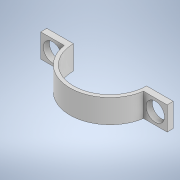
# Autodesk Inventor part: clamphalf
Saved by Autodesk Inventor 2020.2 (Build 242310000, 310)
## iProperties
Created: 2020-02-20
Part Number: clamphalf
Material: Generic
Document SubType Name: Modeling
Designer: ColinP
Density: 1 g/cm^3
Appearance: Default
Author: ColinP
Autodesk Inventor part; units mm, degrees
ref_plane "YZ Plane" through (0, 0, 0) normal (1, 0, 0) x (0, 1, 0)
ref_plane "XZ Plane" through (0, 0, 0) normal (0, 1, 0) x (-1, 0, 0)
ref_plane "XY Plane" through (0, 0, 0) normal (0, 0, 1) x (1, 0, 0)
sketch "Sketch1" plane through (0, 0, 0) normal (0, 1, 0) x (-1, 0, 0)
  circle A0 centre (0, 0) radius 7.75
  circle A1 centre (0, 0) radius 8.5
  line L0 (8.5, 0) -> (7.75, 0)
  line L1 (-7.75, 0) -> (-8.5, 0)
  line L2 (8.5, 0) -> (8.4, 0)
  line L3 (8.4, 0) -> (8.4, 1.3)
  line L4 (8.4, 1.3) -> (13.4, 1.3)
  line L5 (13.4, 1.3) -> (13.4, 0)
  line L6 (13.4, 0) -> (8.5, 0)
  line L7 (-8.5, 0) -> (-8.4, 0)
  line L8 (-8.4, 0) -> (-8.4, 1.3)
  line L9 (-8.4, 1.3) -> (-13.4, 1.3)
  line L10 (-13.4, 1.3) -> (-13.4, 0)
  line L11 (-13.4, 0) -> (-8.5, 0)
  dimension "d0" = 15.5
  dimension "d1" = 17
  dimension "d2" = 0.1
  dimension "d3" = 5
  dimension "d4" = 0.1
  dimension "d5" = 5
  constraints: 24 end point, 8 point on line, 6 point on circle, 5 perpendicular, 2 centre point, 2 coincident, 2 horizontal
  measures "d0" diameter of A0
  measures "d1" diameter of A1
  measures "d2" distance of L0.start L2.end
  measures "d3" distance of L3.end L4.end
  measures "d4" distance of L1.end L7.end
  measures "d5" distance of L8.end L9.end
extrude "Extrusion1" add sketch "Sketch1" along normal blind 5 contours A0 L1 L8 A1 L3 L0 | L3 A1 L0 | L1 A1 L8 | A1 L4 L5 L6 | L11 L10 L9 A1
sketch "Sketch2" plane through (-13.4, 0, 1.3) normal (0, 0, 1) x (1, 0, 0)
  line L0 (5.65, 0) -> (5.65, 5) projected
  line L1 (5.65, 5) -> (5.65, 2.5)
  line L2 (0, 0) -> (0, 5) projected
  line L3 (0, 2.5) -> (2.5, 2.5)
  line L4 (26.8, 0) -> (26.8, 5) projected
  line L5 (26.8, 2.5) -> (24.3, 2.5)
  point P0 (13.4, 0)
  dimension "d8" = 2.5
  dimension "d9" = 2.5
  constraints: 6 end point, 3 midpoint, 2 horizontal
  measures "d8" distance of L3.start L3.end
  measures "d9" distance of L5.start L5.end
hole "Hole1" at (-10.9, 2.5, 1.3) at (10.9, 2.5, 1.3) direction (0, 0, -1) diameter 3.9 end through all clearance for "Flat Head Machine Screw" size "M3.5" standard "Ansi Metric M Profile"
body "Solid1"
